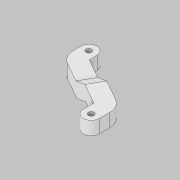
# Autodesk Inventor part: LegConnector
Saved by Autodesk Inventor 2019.2 (Build 232265000, 265)
## iProperties
Created: 2019-02-07
Part Number: LegConnector
Material: ABS-Kunststoff
Document SubType Name: Modeling
Designer: Lion
Density: 1.06 g/cm^3
Appearance: Weiß
Author: Lion
## iProperties of the stored document LegConnector_3D-Druck.ipt
Created: 2019-04-11
Part Number: LegConnector_3D-Druck
Material: Generisch
Document SubType Name: Modeling
Designer: Lion
Density: 1 g/cm^3
Appearance: Vorgabe
Author: Lion
Autodesk Inventor part; units mm, degrees
ref_plane "YZ Plane" through (0, 0, 0) normal (1, 0, 0) x (0, 1, 0)
ref_plane "XZ Plane" through (0, 0, 0) normal (0, 1, 0) x (-1, 0, 0)
ref_plane "XY Plane" through (0, 0, 0) normal (0, 0, 1) x (1, 0, 0)
sketch "Skizze4" plane through (0, 0, 0) normal (0, 1, 0) x (-1, 0, 0)
  arc A0 (3, 0) -> (-3, 0) centre (0, 0) ccw
  line L0 (3, 0) -> (3, -4)
  line L1 (3, -4) -> (-3, -4) construction
  line L2 (-3, -4) -> (-3, 0)
  line L3 (29.4604, -19.0022) -> (26.5011, -24.2217) construction
  line L4 (26.5011, -24.2217) -> (6.9282, -13.1244) construction
  arc A1 (26.5011, -24.2217) -> (29.4604, -19.0022) centre (27.9808, -21.612) ccw construction
  line L5 (0, 0) -> (3, -1.7009) construction
  line L6 (-2.4661, -4.3495) -> (27.9808, -21.612) construction
  line L7 (27.9808, -21.612) -> (30.4468, -17.2624) construction
  line L8 (30.4468, -17.2624) -> (0, 0) construction
  line L9 (0, 0) -> (-2.4661, -4.3495) construction
  line L10 (-2.4661, -4.3495) -> (30.4468, -17.2624) construction
  line L11 (27.9808, -21.612) -> (0, 0) construction
  line L12 (9.8874, -7.905) -> (29.4604, -19.0022) construction
  line L13 (6.9282, -13.1244) -> (0.0407, -9.2195)
  line L14 (9.8874, -7.905) -> (6.9282, -13.1244)
  line L15 (9.8874, -7.905) -> (3, -4)
  arc A2 (-3, -4) -> (0.0407, -9.2195) centre (3, -4) ccw
  point P0 (13.9904, -10.806)
  dimension "d15" = 4
  dimension "d16" = 3
  dimension "d17" = 5
  dimension "d18" = 35
  dimension "d19" = 5
  constraints: 32 end point, 8 parallel, 6 point on circle, 6 tangent, 5 perpendicular, 3 centre point, 2 coincident, 2 midpoint, 1 point on line, 1 vertical
  measures "d15" distance from line of L1 point (0, 0)
  measures "d16" radius of A0
  measures "d17" distance from line of A1.centre L5
  measures "d18" distance from line of point (0, 0) L3
  measures "d19" distance from line of point (13.99, -10.806) L14
extrude "Extrusion4" add sketch "Skizze4" along normal blind 5
sketch "Skizze5" plane through (0, 0, 0) normal (0, -1, 0) x (1, 0, 0)
  line L0 (-9.8874, -7.905) -> (-29.4604, -19.0022) construction
  line L1 (-26.5011, -24.2217) -> (-6.9282, -13.1244) construction
  line L2 (-9.8874, -7.905) -> (-6.9282, -13.1244) projected
  line L3 (-15.6273, -18.0565) -> (-6.9282, -13.1244)
  line L4 (-6.9282, -13.1244) -> (-9.8874, -7.905)
  line L5 (-9.8874, -7.905) -> (-18.5865, -12.8371)
  line L6 (-18.5865, -12.8371) -> (-15.6273, -18.0565)
  line L7 (-15.6273, -18.0565) -> (-9.8874, -7.905) construction
  line L8 (-6.9282, -13.1244) -> (-18.5865, -12.8371) construction
  line L9 (-14.237, -10.371) -> (-11.2777, -15.5905) construction
  point P0 (0, 0)
  point P1 (-13.9904, -10.806)
  point P2 (-12.7573, -12.9808)
  point P3 (-12.7573, -12.9808)
  constraints: 14 end point, 6 midpoint, 2 parallel, 2 perpendicular, 1 point on line
extrude "Extrusion5" add sketch "Skizze5" along normal mid plane 10
sketch "Skizze6" plane through (0, -5, 0) normal (0, -1, 0) x (1, 0, 0)
  line L0 (-9.8874, -7.905) -> (-29.4604, -19.0022) construction
  arc A0 (-26.5011, -24.2217) -> (-29.4604, -19.0022) centre (-27.9808, -21.612) ccw construction
  line L1 (-26.5011, -24.2217) -> (-6.9282, -13.1244) construction
  line L2 (-18.5865, -12.8371) -> (-15.6273, -18.0565) projected
  line L3 (-25.8727, -16.9681) -> (-18.5865, -12.8371)
  line L4 (-15.6273, -18.0565) -> (-22.9134, -22.1876)
  arc A1 (-25.8727, -16.9681) -> (-28.9104, -21.9956) centre (-22.9134, -22.1876) ccw
  line L5 (-27.9808, -21.612) -> (-26.0079, -25.0916) construction
  arc A2 (-29.0064, -24.9956) -> (-23.0094, -25.1876) centre (-26.0079, -25.0916) ccw
  line L6 (-28.9104, -21.9956) -> (-29.0064, -24.9956)
  line L7 (-23.0094, -25.1876) -> (-22.9134, -22.1876)
  point P0 (0, 0)
  dimension "d45" = 4
  dimension "d46" = 3
  constraints: 10 end point, 4 point on circle, 4 tangent, 3 point on line, 2 centre point, 1 coincident, 1 parallel
  measures "d45" distance of L5.start L5.end
  measures "d46" vertical distance of L7.start L4.end
extrude "Extrusion6" add sketch "Skizze6" against normal blind 5
sketch "Skizze7" plane through (0, 0, 0) normal (0, -1, 0) x (1, 0, 0)
  circle A0 centre (0, 0) radius 1.05
  dimension "d26" = 2.1
  constraints: 1 centre point, 1 coincident
  measures "d26" diameter of A0
extrude "Extrusion7" cut sketch "Skizze7" against normal up to next
sketch "Skizze8" plane through (0, -5, 0) normal (0, -1, 0) x (1, 0, 0)
  arc A0 (-29.0064, -24.9956) -> (-23.0094, -25.1876) centre (-26.0079, -25.0916) ccw construction
  circle A1 centre (-26.0079, -25.0916) radius 1.05
  point P0 (0, 0)
  dimension "d47" = 2.1
  constraints: 1 centre point, 1 coincident
  measures "d47" diameter of A1
extrude "Extrusion8" cut sketch "Skizze8" against normal up to next
chamfer "Fase2" distance 9 distance2 5 1 edges at (-17.1069, 5, -15.4468) measured on face at (-7.2091, 5, -8.6855)
chamfer "Fase3" distance 9 distance2 5 1 edges at (-8.4078, -5, -10.5147) measured on face at (-19.5579, -5, -15.6869)
fillet "Rundung2" [suppressed]
